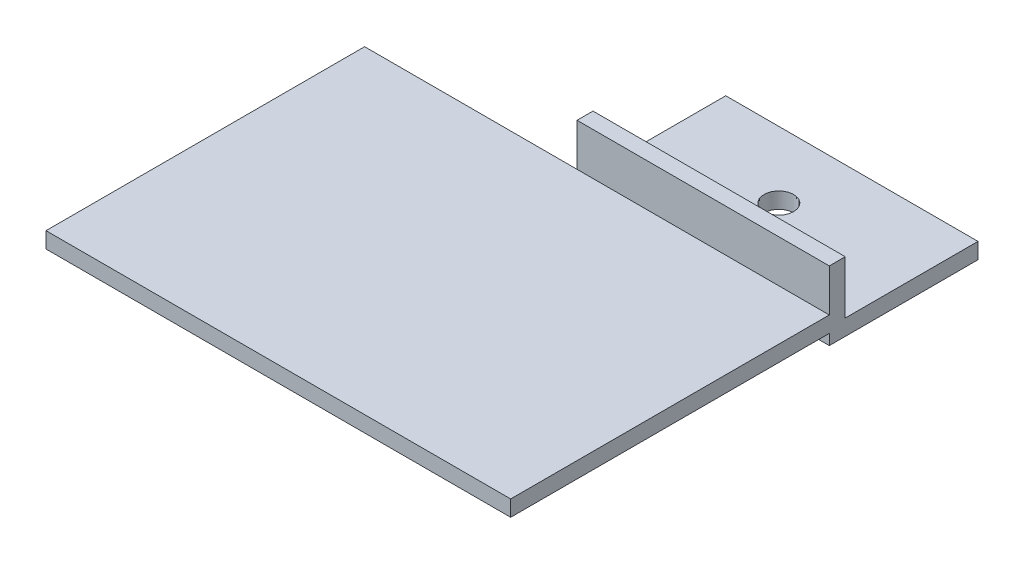
# Autodesk Inventor part: Battery Support
Saved by Autodesk Inventor 2019.4 (Build 234330000, 330)
## iProperties
Created: 2020-03-26
Part Number: Battery Support
Material: PC/ABS Plastic
Document SubType Name: Modeling
Designer: Mark
Mass: 1.90823 g
Surface Area: 41.2652 cm^2
Volume: 5.34111 cm^3
Density: 0.357273 g/cm^3
Appearance: Smooth - White
Author: Mark
Autodesk Inventor part; units mm, degrees
ref_plane "YZ Plane" through (0, 0, 0) normal (1, 0, 0) x (0, 1, 0)
ref_plane "XZ Plane" through (0, 0, 0) normal (0, 1, 0) x (-1, 0, 0)
ref_plane "XY Plane" through (0, 0, 0) normal (0, 0, 1) x (1, 0, 0)
sketch "Sketch1" plane through (0, 0, 0) normal (0, 1, 0) x (-1, 0, 0)
  line L0 (0, 0) -> (47.5, 0)
  line L1 (47.5, 0) -> (47.5, -28)
  line L2 (47.5, -28) -> (0, -28)
  line L3 (0, -28) -> (0, 0)
  dimension "d0" = 47.5
  dimension "d1" = 28
  constraints: 8 end point, 2 parallel, 1 horizontal, 1 perpendicular
  measures "d0" distance of L1.end L2.end
  measures "d1" distance of L0.end L1.end
extrude "Extrusion1" add sketch "Sketch1" along normal blind 3
sketch "Sketch2" plane through (0, 3, 0) normal (0, 1, 0) x (1, 0, 0)
  line L0 (0, 0) -> (0, 28) projected
  line L1 (-47.5, 28) -> (-47.5, 0) projected
  line L2 (0, 0) -> (-47.5, 0)
  line L3 (-47.5, 0) -> (-47.5, 3)
  line L4 (-47.5, 3) -> (0, 3)
  line L5 (0, 3) -> (0, 0)
  dimension "d4" = 3
  constraints: 8 end point, 2 parallel, 1 horizontal, 1 perpendicular, 1 point on line
  measures "d4" distance of L2.end L3.end
extrude "Extrusion2" add sketch "Sketch2" along normal blind 10
sketch "Sketch3" plane through (0, 3, 0) normal (0, 1, 0) x (1, 0, 0)
  circle A0 centre (-25, 15.5) radius 2.8
  line L0 (0, 3) -> (0, 28) projected
  line L1 (0, 28) -> (-47.5, 28) projected
  point P0 (0, 0)
  dimension "d7" = 5.6
  dimension "d8" = 25
  dimension "d9" = 12.5
  constraints: 1 centre point
  measures "d7" diameter of A0
  measures "d8" distance from line of L0 A0.centre
  measures "d9" distance from line of L1 A0.centre
extrude "Extrusion3" cut sketch "Sketch3" against normal blind 10
sketch "Sketch4" plane through (-47.5, 0, 0) normal (0, 0, 1) x (1, 0, 0)
  line L0 (47.5, 0) -> (47.5, 13) projected
  line L1 (0, 0) -> (0, 13) projected
  line L2 (47.5, 2) -> (0, 2)
  line L3 (0, 2) -> (0, 5)
  line L4 (0, 5) -> (47.5, 5)
  line L5 (47.5, 5) -> (47.5, 2)
  line L6 (0, 3) -> (47.5, 3) projected
  dimension "d12" = 3
  dimension "d13" = 1
  constraints: 8 end point, 2 parallel, 2 point on line, 1 horizontal, 1 perpendicular
  measures "d12" distance of L2.end L3.end
  measures "d13" distance between parallel lines of L6 L2
extrude "Extrusion4" add sketch "Sketch4" along normal blind 60
sketch "Sketch5" plane through (-47.5, 0, -28) normal (-1, 0, 0) x (0, 0, 1)
  line L0 (28, 5) -> (88, 5) projected
  line L1 (88, 5) -> (28, 5)
  line L2 (28, 5) -> (28, 2)
  line L3 (28, 2) -> (88, 2)
  line L4 (88, 2) -> (88, 5)
  point P0 (28, 0)
  dimension "d16" = 3
  constraints: 8 end point, 2 parallel, 1 horizontal, 1 perpendicular
  measures "d16" distance of L2.end L1.end
extrude "Extrusion5" add sketch "Sketch5" along normal blind 40
body "Solid1"
